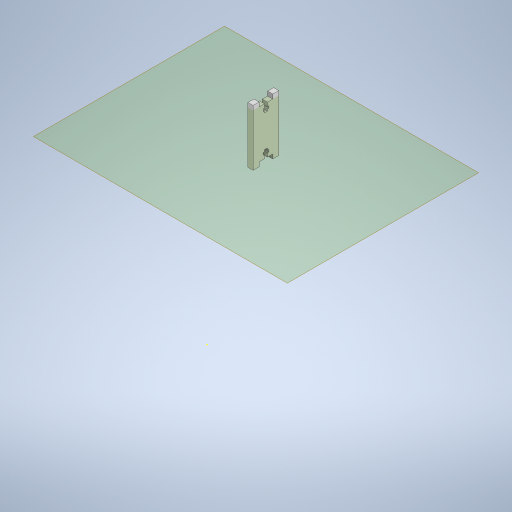
# Autodesk Inventor part: стенка 2
Saved by Autodesk Inventor 2024.2 (Build 282272000, 272)
## iProperties
Created: 2025-12-09
Part Number: стенка 2
Material: Типовые
Document SubType Name: Modeling
Designer: katya_notebook
Density: 1 g/cm^3
Appearance: По умолчанию
Author: katya_notebook
Autodesk Inventor part; units mm, degrees
ref_plane "YZ Plane" through (0, 0, 0) normal (1, 0, 0) x (0, 1, 0)
ref_plane "XZ Plane" through (0, 0, 0) normal (0, 1, 0) x (-1, 0, 0)
ref_plane "XY Plane" through (0, 0, 0) normal (0, 0, 1) x (1, 0, 0)
ref_plane "РабПлоскость1" through (-329.2239, 210.3045, -11.0538) normal (0, -1, 0) x (1, 0, 0)
sketch "Эскиз1" plane through (-329.2239, 210.3045, -11.0538) normal (0, -1, 0) x (1, 0, 0)
  line L0 (-46.5606, -73) -> (-52.5606, -73)
  line L1 (-52.5606, -73) -> (-52.5606, -43)
  line L2 (-52.5606, -43) -> (-46.5606, -43)
  line L3 (-46.5606, -43) -> (-46.5606, -73)
  line L4 (-23.55, -78) -> (-51.55, -78) projected
  point P0 (329.2239, 11.0538)
  dimension "d0" = 6
  dimension "d1" = 30
  dimension "d2" = 5
  constraints: 8 end point, 2 parallel, 1 horizontal, 1 perpendicular
  measures "d0" distance of L1.end L2.end
  measures "d1" distance of L0.end L1.end
  measures "d2" distance from line of L4 L0.start
ref_plane "РабПлоскость2" through (-464.2239, 154.5996, -124.0538) normal (0, 1, 0) x (0, 0, 1)
extrude "Выдавливание1" add sketch "Эскиз1" along normal up to surface (55.705 mm away)
sketch "Эскиз2" plane through (-375.7846, 210.3045, -54.0538) normal (1, 0, 0) x (0, 0, -1)
  line L0 (0, -55.705) -> (30, -55.705) projected
  line L1 (30, -55.705) -> (23, -55.705)
  line L2 (23, -55.705) -> (23, -60.705)
  line L3 (23, -60.705) -> (30, -60.705)
  line L4 (30, -60.705) -> (30, -55.705)
  line L5 (0, -55.705) -> (7, -55.705)
  line L6 (7, -55.705) -> (7, -60.705)
  line L7 (7, -60.705) -> (0, -60.705)
  line L8 (0, -60.705) -> (0, -55.705)
  line L9 (18.25, -51.205) -> (11.75, -51.205)
  line L10 (11.75, -51.205) -> (11.75, -48.705)
  line L11 (11.75, -48.705) -> (18.25, -48.705)
  line L12 (18.25, -48.705) -> (18.25, -51.205)
  line L13 (13.25, -46.5052) -> (16.75, -46.5052)
  line L14 (16.75, -46.5052) -> (16.75, -57.9047)
  line L15 (16.75, -57.9047) -> (13.25, -57.9047)
  line L16 (13.25, -57.9047) -> (13.25, -46.5052)
  line L17 (13.25, -46.5052) -> (16.75, -57.9047) construction
  line L18 (16.75, -46.5052) -> (13.25, -57.9047) construction
  line L19 (30, 0) -> (30, -55.705) projected
  line L20 (30, -27.8525) -> (0, -27.8525)
  line L21 (0, 0) -> (0, -55.705) projected
  line L22 (30, 0) -> (23, 0)
  line L23 (23, 0) -> (23, 5)
  line L24 (23, 5) -> (30, 5)
  line L25 (30, 5) -> (30, 0)
  line L26 (0, 0) -> (7, 0)
  line L27 (7, 0) -> (7, 5)
  line L28 (7, 5) -> (0, 5)
  line L29 (0, 5) -> (0, 0)
  line L30 (18.25, -4.5) -> (11.75, -4.5)
  line L31 (11.75, -4.5) -> (11.75, -7)
  line L32 (11.75, -7) -> (18.25, -7)
  line L33 (18.25, -7) -> (18.25, -4.5)
  line L34 (13.25, -9.1998) -> (16.75, -9.1998)
  line L35 (16.75, -9.1998) -> (16.75, 2.1998)
  line L36 (16.75, 2.1998) -> (13.25, 2.1998)
  line L37 (13.25, 2.1998) -> (13.25, -9.1998)
  line L38 (13.25, -9.1998) -> (16.75, 2.1998) construction
  line L39 (16.75, -9.1998) -> (13.25, 2.1998) construction
  point P0 (-54.0538, -210.3045)
  point P1 (15, -52.205)
  point P2 (7, -55.705)
  point P3 (23, -55.705)
  point P4 (16.75, -51.205)
  point P5 (16.75, -48.705)
  point P6 (13.25, -48.705)
  point P7 (13.25, -51.205)
  point P8 (15, -3.5)
  point P9 (16.75, -7)
  point P10 (16.75, -4.5)
  point P11 (13.25, -4.5)
  point P12 (13.25, -7)
  dimension "d2" = 5
  dimension "d13" = 6.5
  dimension "d14" = 2.5
  dimension "d15" = 5
  dimension "d16" = 7
  dimension "d17" = 4.75
  dimension "d18" = 4.5
  dimension "d19" = 3.5
  dimension "d20" = 3.25
  dimension "d23" = 5
  dimension "d24" = 7
  dimension "d25" = 7
  constraints: 74 end point, 12 parallel, 9 symmetric about line, 6 horizontal, 6 perpendicular, 4 midpoint, 1 collinear, 1 point on line
  measures "d13" distance of L9.start L9.end
  measures "d14" distance of L11.end L9.start
  measures "d15" distance of L3.end L0.end
  measures "d16" distance of L2.end L3.end
  measures "d17" distance between parallel lines of L2 L12
  measures "d18" distance from line of L0 L9.start
  measures "d19" distance of L14.end L15.end
  measures "d20" distance from line of L12 point (15, -52.205)
  measures "d23" distance of L24.end L19.start
  measures "d24" distance of L23.end L24.end
  measures "d25" distance of L27.end L28.end
extrude "Выдавливание2" add sketch "Эскиз2" against normal blind 6 contours L0 L6 L7 L8 | L4 L3 L2 L0 | L22 L23 L24 L25 | L29 L28 L27 L26
sketch "Эскиз3" plane through (-375.7846, 154.5996, -84.0538) normal (1, 0, 0) x (0, 0, -1)
  point P0 (-84.0538, -154.5996)
extrude "Выдавливание3" cut sketch "Эскиз2" against normal blind 6 contours L16 L9 L14 L0 | L0 L14 L15 L16 | L16 L11 L14 L9 | L9 L10 L11 L16 | L14 L11 L12 L9 | L16 L13 L14 L11 | L33 L32 L35 L30 | L35 L32 L37 L30 | L30 L37 L36 L35 | L37 L32 L31 L30 | L35 L34 L37 L32
